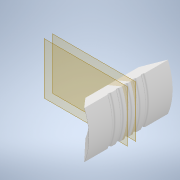
# Autodesk Inventor part: Button
Saved by Autodesk Inventor 2020 (Build 240168000, 168)
## iProperties
Created: 2020-07-05
Part Number: Button
Material: Generic
Document SubType Name: Modeling
Designer: vmiguel
Density: 1 g/cm^3
Appearance: Default
Author: vmiguel
Autodesk Inventor part; units mm, degrees
ref_plane "YZ Plane" through (0, 0, 0) normal (1, 0, 0) x (0, 1, 0)
ref_plane "XZ Plane" through (0, 0, 0) normal (0, 1, 0) x (-1, 0, 0)
sketch "Sketch1" plane through (0, 0, 0) normal (0, 0, 1) x (1, 0, 0)
  circle A0 centre (0, 0) radius 8.25
  circle A1 centre (0, 0) radius 11
  line L0 (0, 0) -> (11, 0) construction
  line L1 (0, 0) -> (10.1627, 4.2095)
  line L2 (0, 0) -> (10.1627, -4.2095)
  point P0 (7.622, -3.1571)
  point P1 (7.622, 3.1571)
  dimension "d0" = 16.5
  dimension "d1" = 22
  dimension "d2" = 45
  dimension "d3" = 22.5
  constraints: 6 end point, 3 point on circle, 2 centre point, 2 coincident, 1 horizontal
  measures "d0" diameter of A0
  measures "d1" diameter of A1
  measures "d2" angle of L2 L1
  measures "d3" angle of L2 L0
extrude "Extrusion1" add sketch "Sketch1" along normal mid plane 11 contours A0 L1 A1 L2 picked at (9.47, 3.4045)
chamfer "Chamfer1" distance 2.7 angle 45 2 edges at (8.25, 0, 5.5) (8.25, 0, -5.5)
sketch "Sketch2" plane through (0, 0, 0) normal (0, 1, 0) x (-1, 0, 0)
  line L0 (-11, -5.5) -> (-11, 5.5) projected
  circle A0 centre (-11, 0) radius 0.25
  line L1 (0, -10.5) -> (0, 10.5) projected
  point P0 (0, 0)
  dimension "d9" = 0.5
  constraints: 1 centre point, 1 midpoint
  measures "d9" diameter of A0
revolve "Revolution1" cut sketch "Sketch2" angle 360 about axis through (0, 0, -10) along (0, 0, 1)
fillet "Fillet1" radius 0.25 4 edges at (10.7886, -2.146, 0.25) (10.7886, 2.146, 0.25) (10.7886, 2.146, -0.25) (10.7886, -2.146, -0.25)
pattern_linear "Rectangular Pattern1" count 3 spacing 1.5 along (0, 0, -1) of "Revolution1", "Fillet1"
pattern_linear "Rectangular Pattern2" count 3 spacing 1.5 along (0, 0, 1) of "Revolution1", "Fillet1"
ref_plane "Work Plane1" through (0, 0, 0.75) normal (0, 0, 1) x (1, 0, 0)
ref_plane "Work Plane2" through (0, 0, -0.75) normal (0, 0, 1) x (1, 0, 0)
sketch "Sketch3" plane through (0, 0, 0.75) normal (0, 0, 1) x (1, 0, 0)
  arc A0 (7.622, -3.1571) -> (7.622, 3.1571) centre (0, 0) ccw projected
  line L0 (5, 1) -> (5, -1)
  line L1 (5, 1) -> (7.9821, 2.0854)
  line L2 (5, -1) -> (7.9821, -2.0854)
  point P0 (5, 0)
  dimension "d20" = 2
  dimension "d21" = 5
  dimension "d22" = 40
  constraints: 6 end point, 2 point on circle, 1 equal length, 1 horizontal alignment, 1 midpoint, 1 vertical
  measures "d20" distance of L0.start L0.end
  measures "d21" distance from line of L0 point (0, 0)
  measures "d22" angle of L2 L1
extrude "Extrusion2" add sketch "Sketch3" along normal blind 2
sketch "Sketch4" plane through (0, 0, -0.75) normal (0, 0, 1) x (1, 0, 0)
  line L0 (7.9821, 2.0854) -> (5, 1) projected
  arc A0 (7.9821, -2.0854) -> (7.9821, 2.0854) centre (0, 0) ccw projected
  line L1 (5, -1) -> (7.9821, -2.0854) projected
  line L2 (5, 1) -> (5, -1) projected
extrude "Extrusion3" add sketch "Sketch4" against normal blind 2
fillet "Fillet2" radius 0.25 2 edges at (5, 0, 0.75) (5, 0, -0.75)
equation "\"d3\" = 0.5 * d2"
body "Solid1"
